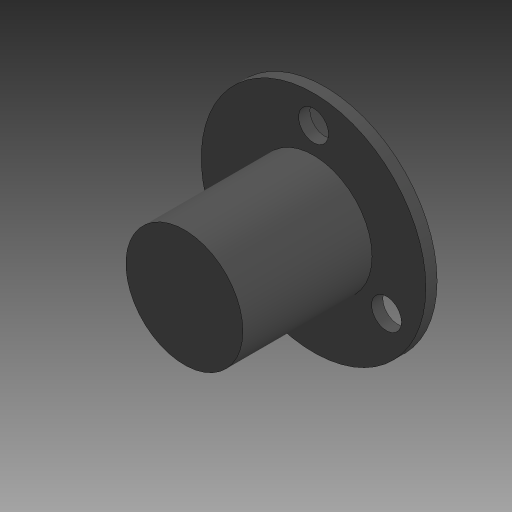
# Autodesk Inventor part: OtocnaKontaktniPruchodka
Saved by Autodesk Inventor 2023 (Build 270158000, 158)
## iProperties
Created: 2024-02-02
Part Number: OtocnaKontaktniPruchodka
Material: Všeobecné
Document SubType Name: Modeling
Designer: matej
Mass: 2.21332 g
Surface Area: 15.2983 cm^2
Volume: 2.21332 cm^3
Density: 1 g/cm^3
Appearance: Všeobecné
Author: matej
Autodesk Inventor part; units mm, degrees
ref_plane "YZ Plane" through (0, 0, 0) normal (1, 0, 0) x (0, 1, 0)
ref_plane "XZ Plane" through (0, 0, 0) normal (0, 1, 0) x (-1, 0, 0)
ref_plane "XY Plane" through (0, 0, 0) normal (0, 0, 1) x (1, 0, 0)
sketch "Náčrt1" plane through (0, 0, 0) normal (0, 0, 1) x (1, 0, 0)
  circle A0 centre (0, 0) radius 12
  dimension "d0" = 24
  constraints: 1 centre point, 1 coincident
  measures "d0" diameter of A0
extrude "Vysunutí1" add sketch "Náčrt1" along normal blind 1.2
sketch "Náčrt2" plane through (0, 0, 1.2) normal (0, 0, 1) x (1, 0, 0)
  circle A0 centre (0, 0) radius 9 construction
  circle A1 centre (0, 9) radius 1.6
  circle A2 centre (-7.7942, -4.5) radius 1.6
  circle A3 centre (7.7942, -4.5) radius 1.6
  dimension "d3" = 18
  dimension "d4" = 3.2
  dimension "d7" = 360
  constraints: 3 centre point, 1 coincident, 1 vertical alignment, 9 other
  measures "d4" diameter of A1
extrude "Vysunutí2" cut sketch "Náčrt2" against normal through all
sketch "Náčrt3" plane through (0, 0, 1.2) normal (0, 0, 1) x (1, 0, 0)
  circle A0 centre (0, 0) radius 6.25
  dimension "d11" = 12.5
  constraints: 1 centre point, 1 coincident
  measures "d11" diameter of A0
extrude "Vysunutí3" add sketch "Náčrt3" along normal blind 13.8
sketch "Náčrt4" plane through (0, 0, 0) normal (0, 0, -1) x (-1, 0, 0)
  circle A0 centre (0, 0) radius 2.5
  dimension "d14" = 5
  constraints: 1 centre point, 1 coincident
  measures "d14" diameter of A0
extrude "Vysunutí4" add sketch "Náčrt4" along normal blind 0.3
